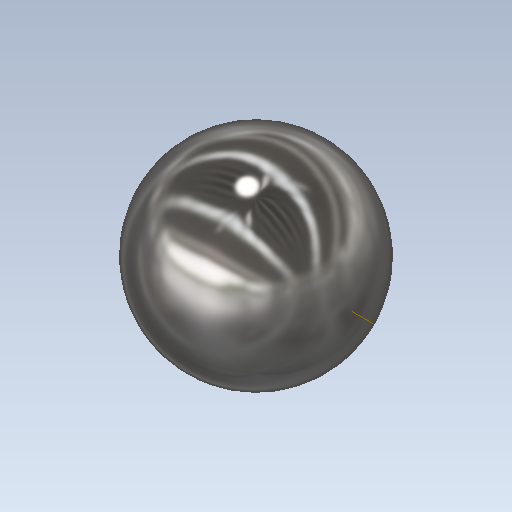
# Autodesk Inventor part: BearingBall
Saved by Autodesk Inventor 2020 (Build 240168000, 168)
## iProperties
Created: 2019-05-05
Part Number: BearingBall
Material: Stal nierdzewna
Document SubType Name: Modeling
Designer: barto
Density: 8 g/cm^3
Appearance: Częściowo polerowana
Author: barto
Autodesk Inventor part; units mm, degrees
ref_plane "YZ Plane" through (0, 0, 0) normal (1, 0, 0) x (0, 1, 0)
ref_plane "XZ Plane" through (0, 0, 0) normal (0, 1, 0) x (-1, 0, 0)
sketch "Szkic1" plane through (0, 0, 0) normal (0, 1, 0) x (-1, 0, 0)
  arc A0 (-3, 0) -> (3, 0) centre (0, 0) ccw
  line L0 (3, 0) -> (-3, 0)
  dimension "d0" = 6
  constraints: 2 end point, 2 point on circle, 1 centre point, 1 coincident
  measures "d0" diameter of A0
revolve "Obrót1" add sketch "Szkic1" angle 360 about axis through (-3, 0, 0) along (1, 0, 0)
ref_plane "Płaszczyzna konstrukcyjna1" through (-3, 0, 0) normal (-1, 0, 0) x (0, -1, 0)
